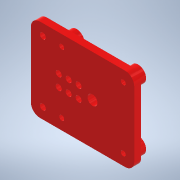
# Autodesk Inventor part: housing
Saved by Autodesk Inventor 2020 (Build 240168000, 168)
## iProperties
Created: 2020-02-03
Part Number: housing
Material: PET Plastic
Document SubType Name: Modeling
Designer: Felix
Density: 1.541 g/cm^3
Appearance: Smooth - Red
Author: Felix
Autodesk Inventor part; units mm, degrees
ref_plane "YZ Plane" through (0, 0, 0) normal (1, 0, 0) x (0, 1, 0)
ref_plane "XZ Plane" through (0, 0, 0) normal (0, 1, 0) x (-1, 0, 0)
ref_plane "XY Plane" through (0, 0, 0) normal (0, 0, 1) x (1, 0, 0)
sketch "Sketch1" plane through (0, 0, 0) normal (0, 0, 1) x (1, 0, 0)
  circle A0 centre (-15.5, -15.5) radius 1.2295 construction
  circle A1 centre (15.5, 15.5) radius 1.2295 construction
  circle A2 centre (15.5, -15.5) radius 1.2295 construction
  circle A3 centre (-15.5, 15.5) radius 1.2295 construction
  circle A4 centre (0, 0) radius 11 construction
  arc A5 (-16.5, 21) -> (-21, 16.5) centre (-16.5, 16.5) ccw construction
  line L0 (-21, 16.5) -> (-21, -16.5) construction
  arc A6 (-21, -16.5) -> (-16.5, -21) centre (-16.5, -16.5) ccw construction
  line L1 (-16.5, -21) -> (16.5, -21) construction
  arc A7 (16.5, -21) -> (21, -16.5) centre (16.5, -16.5) ccw construction
  line L2 (21, -16.5) -> (21, 16.5) construction
  arc A8 (21, 16.5) -> (16.5, 21) centre (16.5, 16.5) ccw construction
  line L3 (16.5, 21) -> (-16.5, 21) construction
  line L4 (16.5, 21) -> (-26.5, 21)
  line L5 (-31, 16.5) -> (-31, -16.5)
  line L6 (-26.5, -21) -> (16.5, -21)
  line L7 (21, -16.5) -> (21, 16.5)
  arc A9 (21, 16.5) -> (16.5, 21) centre (16.5, 16.5) ccw
  arc A10 (16.5, -21) -> (21, -16.5) centre (16.5, -16.5) ccw
  arc A11 (-31, -16.5) -> (-26.5, -21) centre (-26.5, -16.5) ccw
  arc A12 (-26.5, 21) -> (-31, 16.5) centre (-26.5, 16.5) ccw
  circle A13 centre (15.5, 15.5) radius 1.2295
  circle A14 centre (15.5, -15.5) radius 1.2295
  circle A15 centre (-15.5, -15.5) radius 1.2295
  circle A16 centre (-15.5, 15.5) radius 1.2295
  circle A17 centre (0, 0) radius 11 construction
  circle A18 centre (0, 0) radius 5 construction
  circle A19 centre (0, 0) radius 10 construction
  circle A20 centre (0, 0) radius 15 construction
  line L8 (-7, 3) -> (-7, -3) construction
  line L9 (-12, 3) -> (-12, -3) construction
  line L10 (-17, 3) -> (-17, -3) construction
  circle A21 centre (-7, 3) radius 1.5
  circle A22 centre (-7, -3) radius 1.5
  circle A23 centre (-12, 3) radius 1.5
  circle A24 centre (-12, -3) radius 1.5
  circle A25 centre (-17, 3) radius 1.5
  circle A26 centre (-17, -3) radius 1.5
  circle A27 centre (-25, 15.5) radius 1.5
  circle A28 centre (-25, -15.5) radius 1.5
  circle A29 centre (0, 0) radius 2.5
  point P0 (-7, 0)
  point P1 (-12, 0)
  point P2 (-17, 0)
  point P3 (-5, 0)
  point P4 (-10, 0)
  point P5 (-15, 0)
  point P6 (-10.5169, -3.2242)
  point P7 (-10.7969, -2.1042)
  point P8 (-10.7969, 2.1042)
  point P9 (-10.5169, 3.2242)
extrude "Extrusion1" add sketch "Sketch1" along normal blind 3.5
sketch "Sketch3" plane through (0, 0, 0) normal (0, 0, -1) x (-1, 0, 0)
  circle A0 centre (-15.5, 15.5) radius 1.2295 projected
  circle A1 centre (15.5, 15.5) radius 1.2295 projected
  circle A2 centre (15.5, -15.5) radius 1.2295 projected
  circle A3 centre (-15.5, -15.5) radius 1.2295 projected
  circle A4 centre (-15.5, 15.5) radius 4
  circle A5 centre (15.5, 15.5) radius 4
  circle A6 centre (15.5, -15.5) radius 4
  circle A7 centre (-15.5, -15.5) radius 4
  point P0 (0, 0)
  dimension "d37" = 8
  dimension "d38" = 8
  dimension "d39" = 8
  dimension "d40" = 8
  constraints: 4 centre point, 4 coincident
  measures "d37" diameter of A4
  measures "d38" diameter of A5
  measures "d39" diameter of A6
  measures "d40" diameter of A7
extrude "Extrusion2" add sketch "Sketch3" along normal blind 4
equation "\"d38\" = d37"
equation "\"d39\" = d37"
equation "\"d40\" = d37"
equation "\"d6\" = d5"
equation "\"d7\" = d5"
equation "\"d5\" = 6"
body "Solid1"
